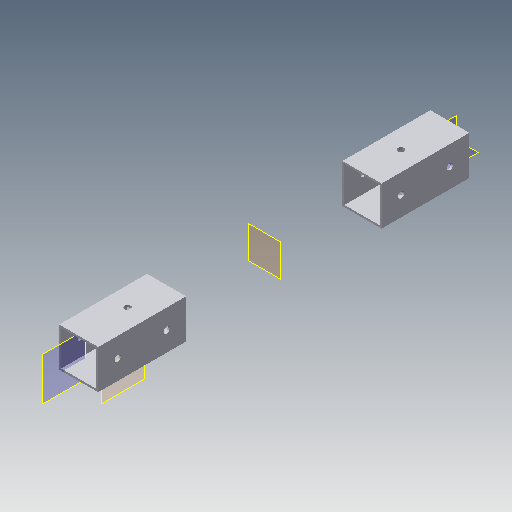
# Autodesk Inventor part: ロボベース□15
Saved by Autodesk Inventor 2019.4 (Build 234330000, 330)
## iProperties
Created: 2018-08-09
Part Number: ロボベース□15
Material: 一般
Document SubType Name: Modeling
Designer: Owner
Density: 1 g/cm^3
Appearance: 既定
Mass: 6.74349 g
Surface Area: 139.116 cm^2
Volume: 6.74349 cm^3
Author: Owner
Autodesk Inventor part; units mm, degrees
ref_plane "YZ Plane" through (0, 0, 0) normal (1, 0, 0) x (0, 1, 0)
ref_plane "XZ Plane" through (0, 0, 0) normal (0, 1, 0) x (-1, 0, 0)
ref_plane "XY Plane" through (0, 0, 0) normal (0, 0, 1) x (1, 0, 0)
ref_plane "作業平面2" through (7.5, -7.5, 160) normal (1, 0, 0) x (0, 0, -1)
ref_plane "作業平面1" through (7.5, -7.5, 80) normal (0, 0, 1) x (1, 0, 0)
sketch "スケッチ2" plane through (7.5, -7.5, 80) normal (0, 0, 1) x (1, 0, 0)
  line L0 (-17.5, 17.5) -> (2.5, 17.5)
  line L1 (2.5, 17.5) -> (2.5, -2.5)
  line L2 (2.5, -2.5) -> (-17.5, -2.5)
  line L3 (-17.5, -2.5) -> (-17.5, 17.5)
  line L4 (-17.5, 17.5) -> (2.5, -2.5) construction
  line L5 (2.5, 17.5) -> (-17.5, -2.5) construction
  point P0 (-7.5, 7.5)
  dimension "d4" = 20
  dimension "d5" = 20
  constraints: 12 end point, 2 midpoint, 2 parallel, 1 horizontal, 1 perpendicular
  measures "d4" distance of L1.end L2.end
  measures "d5" distance of L0.end L1.end
extrude "押し出し2" add sketch "スケッチ2" along normal mid plane 190
shell "シェル1" thickness 1 removed faces 2 at (3.3333, -3.3333, 175) at (-3.3333, 3.3333, -15)
ref_plane "作業平面3" through (-7.5, -7.5, -15) normal (-1, 0, 0) x (0, 0, 1)
sketch "スケッチ3" plane through (-10, -7.5, -15) normal (-1, 0, 0) x (0, 0, 1)
  line L0 (155, 7.5) -> (35, 7.5)
  line L1 (190, -2.5) -> (0, -2.5) projected
  line L2 (190, 17.5) -> (190, -2.5) projected
  point P0 (95, -2.5)
  point P1 (95, 7.5)
  point P2 (190, 7.5)
  dimension "d38" = 120
  constraints: 3 midpoint, 2 end point, 1 horizontal, 1 horizontal alignment, 1 vertical alignment
  measures "d38" distance of L0.start L0.end
hole "穴1" at (-10, 0, 140) at (-10, 0, 20) direction (1, 0, 0) diameter 3.2 end through all
ref_plane "作業平面4" through (-7.5, -7.5, -15) normal (0, -1, 0) x (1, 0, 0)
sketch "スケッチ4" plane through (-7.5, -10, -15) normal (0, -1, 0) x (1, 0, 0)
  line L0 (17.5, 190) -> (17.5, 0) projected
  line L1 (-2.5, 190) -> (17.5, 190) projected
  line L2 (-2.5, 190) -> (-2.5, 0) projected
  line L3 (17.5, 0) -> (-2.5, 0) projected
  line L4 (7.5, 165) -> (7.5, 25)
  line L5 (17.5, 190) -> (17.5, 0) projected
  line L6 (-2.5, 190) -> (17.5, 190) projected
  point P0 (17.5, 95)
  point P1 (7.5, 95)
  point P2 (7.5, 190)
  dimension "d39" = 140
  constraints: 3 midpoint, 2 end point, 1 horizontal alignment, 1 parallel, 1 vertical alignment
  measures "d39" distance of L4.start L4.end
hole "穴2" at (0, -10, 150) at (0, -10, 10) direction (0, 1, 0) diameter 3.2 end through all
sketch "スケッチ5" plane through (7.5, -7.5, 80) normal (0, 0, 1) x (1, 0, 0)
  line L0 (2.5, 17.5) -> (-17.5, 17.5)
  line L1 (-17.5, 17.5) -> (-17.5, -2.5)
  line L2 (-17.5, -2.5) -> (2.5, -2.5)
  line L3 (2.5, -2.5) -> (2.5, 17.5)
  line L4 (2.5, 17.5) -> (-17.5, -2.5) construction
  line L5 (-17.5, 17.5) -> (2.5, -2.5) construction
  point P0 (-7.5, 7.5)
  dimension "d25" = 20
  dimension "d26" = 20
  constraints: 12 end point, 2 midpoint, 2 parallel, 1 horizontal, 1 perpendicular
  measures "d25" distance of L2.end L1.end
  measures "d26" distance of L1.end L0.end
extrude "押し出し3" cut sketch "スケッチ5" along normal mid plane 100
ref_plane "作業平面5" through (-7.5, -7.5, 175) normal (-1, 0, 0) x (0, 0, 1)
sketch "スケッチ6" plane through (-10, -7.5, 175) normal (-1, 0, 0) x (0, 0, 1)
  line L0 (-45, 17.5) -> (-45, -2.5) projected
  line L1 (0, -2.5) -> (-45, -2.5) projected
  line L2 (0, 17.5) -> (0, -2.5) projected
  line L3 (-45, 17.5) -> (0, 17.5) projected
  circle A0 centre (-35, 7.5) radius 1.6 projected
  circle A1 centre (-155, 7.5) radius 1.6 projected
  line L4 (-145, -2.5) -> (-145, 17.5) projected
  line L5 (-190, 17.5) -> (-145, 17.5) projected
  line L6 (-190, -2.5) -> (-190, 17.5) projected
  line L7 (-145, -2.5) -> (-190, -2.5) projected
  line L8 (-10, 7.5) -> (-180, 7.5)
  line L9 (0, 17.5) -> (0, -2.5) projected
  line L10 (-190, -2.5) -> (-190, 17.5) projected
  point P0 (0, 7.5)
  dimension "d40" = 10
  dimension "d41" = 10
  constraints: 2 end point, 1 horizontal, 1 midpoint, 1 point on line
  measures "d40" distance from line of L9 L8.start
  measures "d41" distance from line of L10 L8.end
hole "穴3" at (-10, 0, 165) at (-10, 0, -5) direction (1, 0, 0) diameter 3.2 end through all
equation "\"d5\" = d4"
equation "\"d26\" = d25"
